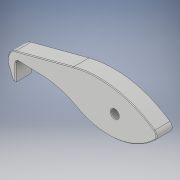
# Autodesk Inventor part: Součást22
Saved by Autodesk Inventor 2019 (Build 230136000, 136)
## iProperties
Created: 2020-01-21
Part Number: Součást22
Material: Všeobecné
Document SubType Name: Modeling
Designer: hynek
Density: 1 g/cm^3
Appearance: Výchozí
Author: hynek
Autodesk Inventor part; units mm, degrees
ref_plane "YZ Plane" through (0, 0, 0) normal (1, 0, 0) x (0, 1, 0)
ref_plane "XZ Plane" through (0, 0, 0) normal (0, 1, 0) x (-1, 0, 0)
ref_plane "XY Plane" through (0, 0, 0) normal (0, 0, 1) x (1, 0, 0)
sketch "Náčrt1" plane through (0, 0, 0) normal (0, 0, 1) x (1, 0, 0)
  line L0 (-106.433, 0) -> (55.3696, 0) projected
  line L1 (0, -81.7425) -> (0, 52.651) projected
  circle A0 centre (0, 0) radius 3
  arc A1 (30.8349, -1.8219) -> (30.2938, 4.277) centre (28, 1) ccw
  arc A2 (-76.0338, 3.7372) -> (-82, -4) centre (-74, -4) ccw
  arc A3 (-73.9347, -2.0011) -> (-75.9978, -4.0942) centre (-74, -4) ccw
  line L2 (-75.9978, -3.9058) -> (-75.9978, -16.9058)
  line L3 (-75.9978, -16.9058) -> (-77.9978, -16.9058)
  line L4 (-77.9978, -16.9058) -> (-82, -7)
  line L5 (-82, -4) -> (-82, -7)
  arc A4 (30.2938, 4.277) -> (-31.7818, 15.3695) centre (-12.7146, -57.1663) ccw
  arc A5 (-29.0159, -10.1823) -> (30.8349, -1.8219) centre (-4.6017, 33.4519) ccw
  arc A6 (-29.0159, -10.1823) -> (-56.3536, -2.5755) centre (-58.3128, -62.5435) ccw
  line L6 (-76.0338, 3.7372) -> (-31.7818, 15.3695)
  line L7 (-73.9347, -2.0011) -> (-56.3536, -2.5755)
  dimension "d0" = 6
  dimension "d1" = 8
  dimension "d2" = 28
  dimension "d3" = 1
  dimension "d4" = 16
  dimension "d5" = 4
  dimension "d6" = 4
  dimension "d7" = 74
  dimension "d8" = 13
  dimension "d9" = 158
  dimension "d10" = 2
  dimension "d11" = 3
  dimension "d12" = 75
  dimension "d13" = 50
  dimension "d14" = 60
  constraints: 13 point on circle, 12 end point, 8 tangent, 7 centre point, 2 coincident, 2 vertical, 1 horizontal, 1 point on line
  measures "d0" diameter of A0
  measures "d1" diameter of A1
  measures "d2" horizontal distance of A0.centre A1.centre
  measures "d3" distance from line of L0 A1.centre
  measures "d4" diameter of A2
  measures "d5" diameter of A3
  measures "d6" distance from line of L0 A2.centre
  measures "d7" distance from line of L1 A2.centre
  measures "d8" distance of L2.start L2.end
  measures "d9" angle of L5 L4
  measures "d10" distance of L2.end L3.end
  measures "d11" distance of L5.start L4.end
  measures "d12" radius of A4
  measures "d13" radius of A5
  measures "d14" radius of A6
extrude "Vysunutí1" add sketch "Náčrt1" along normal blind 12 contours A2 L6 A4 L1 A0 L0 | L0 A0 L1 A5 A6 L7 A3 L2 L3 L4 L5 A2 | L1 A4 A1 L0 A0 | A0 L0 A1 A5 L1
chamfer "Zkosení1" distance 0.5 angle 45 15 edges at (-79.9989, -11.9529, 12) (-76.9978, -16.9058, 12) (-75.9978, -10.5, 12) (-76, -4, 12) (-75.3567, -2.5305, 12) (-65.1442, -2.2883, 12) (-42.2286, -4.7395, 12) (2.3155, -16.0673, 12) (31.9843, 1.3535, 12) (0.4784, 16.6642, 12) (-53.9078, 9.5533, 12) (-80.3352, 0.8851, 12) (-82, -5.5, 12) (-3, 0, 12) (-3, 0, 0)
